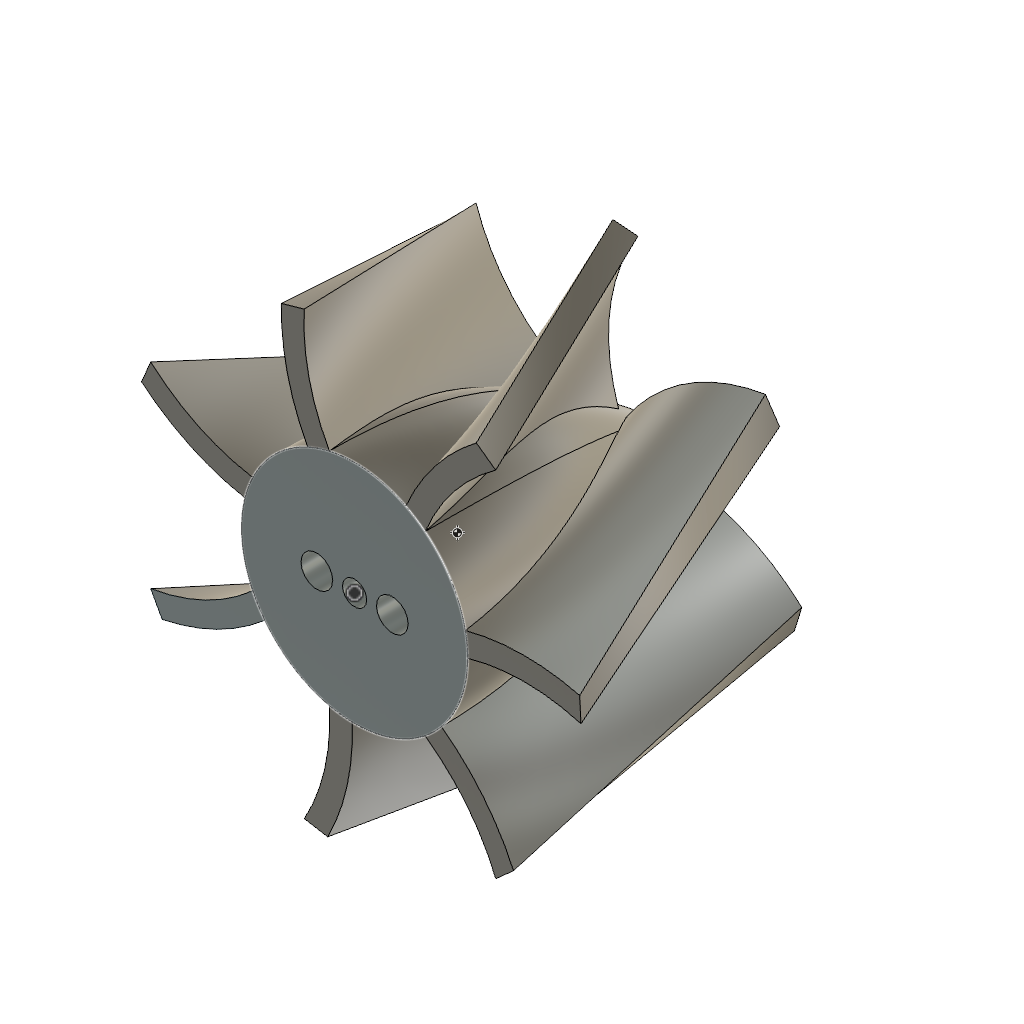
HandFan (Autodesk Fusion 360 archive; units mm, degrees)
design "impeller"
part number: 2026-09-26-12-13-54-947
Autodesk Fusion 360 part; units mm, degrees
sketch "Sketch1" plane through (0, 0, 0) normal (0, 0, 1) x (1, 0, 0)
  line L0 (0, 0) -> (0, 20)
  line L1 (0, 0) -> (7.5, 0)
  spline S0 degree 5 poles (0, 20) (0.4664, 19.4696) (1.3798, 18.3776) (2.6919, 16.6455) (4.3173, 14.135) (6.0412, 10.4977) (7.0187, 6.9371) (7.4124, 3.7167) (7.5, 1.2862) (7.5, 0) knots 0 0 0 0 0 0 0.2 0.4 0.6 0.8 1 1 1 1 1 1
  line L2 (7.5, 3.1786) -> (7.5, -3.1786)
  dimension "d1" = 20
  dimension "d2" = 7.5
  constraint coincident L0.start L1.start
  constraint vertical L0
  constraint perpendicular L0 L1
  constraint midpoint L1.end L2
  measures "d1" distance of L0.start L0.end
  measures "d2" distance of L0.start L1.end
revolve "Revolve1" add sketch "Sketch1" angle 360 about axis through (0, 0, 0) along (0, 1, 0) makes body 1
sketch "Sketch2" plane through (0, 0, 0) normal (0, -1, 0) x (1, 0, 0)
  circle A0 centre (0, 0) radius 7.5
  circle A1 centre (0, 0) radius 0.8
  line L0 (-7.5, 0.0223) -> (7.5, -0.0223)
  circle A2 centre (-2.5, 0) radius 1.05
  circle A3 centre (2.5, -0.0074) radius 1.05
  dimension "d4" = 1.6
  dimension "d5" = 2.1
  dimension "d6" = 2.1
  dimension "d7" = 2.5
  dimension "d8" = 2.5
  constraint coincident A0.centre A1.centre
  constraint coincident A0 L0.start
  constraint coincident A0 L0.end
  constraint perpendicular A0 L0
  constraint coincident L0 A3.centre
  measures "d4" diameter of A1
  measures "d5" diameter of A2
  measures "d6" diameter of A3
  measures "d7" distance of A0.centre A2.centre
  measures "d8" horizontal distance of A0.centre A3.centre
sketch "Sketch3" plane through (0, 0, 0) normal (0, -1, 0) x (1, 0, 0)
  circle A0 centre (0, 0) radius 7.5
  circle A1 centre (0, 0) radius 15
  arc A2 (15, 0) -> (7.5, 0) centre (11.25, -12.8829) ccw
  arc A3 (15.4192, 1.4402) -> (7.0808, 1.4402) centre (11.25, -12.8829) ccw
  line L0 (7.3455, 1.5146) -> (7.5, 0)
  line L1 (14.9169, 1.577) -> (15, 0)
  dimension "d11" = 30
  dimension "d12" = 1.5
  constraint coincident A0.centre A1.centre
  constraint coincident A0 A2.end
  constraint coincident A1 A2.start
  constraint coincident A0 L0.start
  constraint coincident A3 L0.start
  constraint coincident A3 L1.start
  constraint coincident A1 L1.start
  measures "d11" diameter of A1
ref_plane "WorkPlane1" through (11.1727, 17, 1.2695) normal (0, -1, 0) x (1, 0, 0)
sketch "Sketch5" plane through (0, 17, 0) normal (0, -1, 0) x (-1, 0, 0)
sketch "Sketch6" plane through (0, 17, 0) normal (0, -1, 0) x (-1, 0, 0)
  arc A0 (-7.1187, -0.9343) -> (-2.12, -1.05) centre (-4.5026, 4.0523) ccw
  arc A1 (-12.8512, -1.9155) -> (-11.1751, -6.6262) centre (0.2402, 0.0889) ccw
  arc A2 (-11.1751, -6.6262) -> (-2.12, -1.05) centre (-12.3662, 5.4484) ccw
  arc A3 (-12.2849, -8.1846) -> (-0.3524, -0.9962) centre (-12.3662, 5.4484) ccw
  line L0 (-2.12, -1.05) -> (-1.0294, -2.1239)
  line L1 (-11.1751, -6.6262) -> (-10.2306, -8.0165)
  dimension "d16" = 5
  dimension "d17" = 5
  dimension "d18" = 1.5
  constraint coincident A3 L0.end
  constraint coincident A3 L1.end
  measures "d16" distance of A0.start A0.end
  measures "d17" distance of A1.start A1.end
sketch "Sketch7" plane through (0, 0, 0) normal (0, -1, 0) x (1, 0, 0)
loft "Loft1" add profiles "Sketch3", "Sketch6" section 1 contours A0 A2 A3 L1 section 2 bodies 1
pattern_circular "C-Pattern1" count 7 over 360 about axis through (0, 1.75, 0) along (0, 1, 0) of bodies 1 makes body 2 at (9.0018, 10.1717, -3.6116) makes body 3 at (2.7889, 10.1717, -9.2896) makes body 4 at (-5.5241, 10.1717, -7.9724) makes body 5 at (-9.6773, 10.1717, -0.6518) makes body 6 at (-6.5433, 10.1717, 7.1596) makes body 7 at (1.518, 10.1717, 9.5797)
sketch "Sketch8" plane through (0, 0, 0) normal (0, -1, 0) x (1, 0, 0)
  arc A0 (-5.9609, -4.5517) -> (-6.7573, -3.2541) centre (0, 0) ccw
  arc A1 (-13.5145, -6.5083) -> (-6.7573, -3.2541) centre (-15.7256, 6.7259) ccw
  line L0 (-13.5145, -6.5083) -> (-12.7554, -7.893)
  arc A2 (-12.7554, -7.893) -> (-5.9609, -4.5517) centre (-15.7256, 6.7259) ccw
  circle A3 centre (0, 0) radius 7.5
  dimension "d21" = 15
  constraint coincident A0.centre A3.centre
  measures "d21" diameter of A3
sketch "Sketch9" plane through (0, 0, 0) normal (0, -1, 0) x (1, 0, 0)
  circle A0 centre (0, 0) radius 0.8
  line L0 (-7.5, 0) -> (7.5, 0)
  circle A1 centre (-2.5, 0) radius 1.05
  circle A2 centre (2.5, 0) radius 1.05
  dimension "d22" = 1.6
  dimension "d23" = 2.1
  dimension "d24" = 2.1
  dimension "d25" = 2.5
  dimension "d26" = 2.5
  constraint coincident A0.centre origin
  constraint horizontal L0
  constraint coincident L0 A1.centre
  constraint coincident L0 A2.centre
  measures "d22" diameter of A0
  measures "d23" diameter of A1
  measures "d24" diameter of A2
  measures "d25" distance of A0.centre A1.centre
  measures "d26" distance of A0.centre A2.centre
extrude "Extrude2" cut sketch "Sketch9" against normal blind 4 bodies 1 2 3 4 5 6 7
